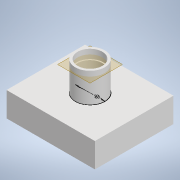
# Autodesk Inventor part: BrakeCover
Saved by Autodesk Inventor 2021 (Build 250183000, 183)
## iProperties
Created: 2021-03-19
Part Number: BrakeCover
Material: Generic
Document SubType Name: Modeling
Designer: ben
Density: 1 g/cm^3
Appearance: Default
Author: ben
Autodesk Inventor part; units mm, degrees
ref_plane "YZ Plane" through (0, 0, 0) normal (1, 0, 0) x (0, 1, 0)
ref_plane "XZ Plane" through (0, 0, 0) normal (0, 1, 0) x (-1, 0, 0)
ref_plane "XY Plane" through (0, 0, 0) normal (0, 0, 1) x (1, 0, 0)
sketch "Sketch2" plane through (0, 0, 0) normal (0, 1, 0) x (-1, 0, 0)
  line L0 (90, -80) -> (-90, -80)
  line L1 (-90, -80) -> (-90, 80)
  line L2 (-90, 80) -> (90, 80)
  line L3 (90, 80) -> (90, -80)
  line L4 (90, -80) -> (-90, 80) construction
  line L5 (-90, -80) -> (90, 80) construction
  point P0 (0, 0)
  dimension "d0" = 180
  dimension "d1" = 160
  constraints: 12 end point, 2 midpoint, 2 parallel, 1 horizontal, 1 perpendicular
  measures "d0" distance of L1.end L2.end
  measures "d1" distance of L0.end L1.end
extrude "Extrusion1" add sketch "Sketch2" along normal blind 50
shell "Shell1" thickness 10 removed faces 1 at (30, 0, -26.6667)
sketch "Sketch4" plane through (0, 0, 0) normal (0, -1, 0) x (1, 0, 0)
  line L0 (-80, 70) -> (80, 70) projected
  line L1 (-80, -70) -> (-80, 70) projected
  line L2 (80, -70) -> (-80, -70) projected
  line L3 (80, 70) -> (80, -70) projected
  point P0 (0, 0)
extrude "Extrusion3" add sketch "Sketch4" against normal blind 10 separate body
sketch "Sketch5" plane through (0, 50, 0) normal (0, 1, 0) x (1, 0, 0)
  circle A0 centre (0, 0) radius 25
  circle A1 centre (0, 0) radius 30
  dimension "d9" = 50
  dimension "d10" = 60
  constraints: 2 centre point, 2 coincident
  measures "d9" diameter of A0
  measures "d10" diameter of A1
extrude "Extrusion4" add sketch "Sketch5" along normal blind 60 separate body
extrude "Extrusion5" cut sketch "Sketch5" against normal blind 120 contours A0 bodies 1
ref_plane "Work Plane1" through (0, 100, 0) normal (0, 1, 0) x (1, 0, 0)
sketch "Sketch6" plane through (0, 100, 0) normal (0, 1, 0) x (1, 0, 0)
  circle A0 centre (0, 0) radius 25 projected
  circle A1 centre (0, 0) radius 27.5
  dimension "d16" = 55
  constraints: 1 centre point, 1 coincident
  measures "d16" diameter of A1
extrude "Extrusion6" cut sketch "Sketch6" against normal blind 10 bodies 3
body "Solid3"
